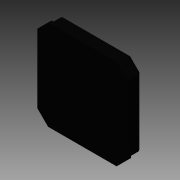
# Autodesk Inventor part: ADAU1761
Saved by Autodesk Inventor 2013 (Build 170138000, 138)
## iProperties
Created: 2015-07-03
Part Number: ADAU1761
Material: Ogólny
Document SubType Name: Modeling
Designer: terg
Density: 1 g/cm^3
Author: terg
Autodesk Inventor part; units mm, degrees
ref_plane "YZ Plane" through (0, 0, 0) normal (1, 0, 0) x (0, 1, 0)
ref_plane "XZ Plane" through (0, 0, 0) normal (0, 1, 0) x (-1, 0, 0)
ref_plane "XY Plane" through (0, 0, 0) normal (0, 0, 1) x (1, 0, 0)
sketch "Szkic1" plane through (0, 0, 0) normal (0, 1, 0) x (-1, 0, 0)
  line L0 (-0.6, 0) -> (-4.4, 0)
  line L1 (-5, -0.6) -> (-5, -4.4)
  line L2 (-4.4, -5) -> (-0.6, -5)
  line L3 (0, -4.4) -> (0, -0.6)
  line L4 (0, -4.4) -> (-0.6, -5)
  line L5 (-4.4, -5) -> (-5, -4.4)
  line L6 (-5, -0.6) -> (-4.4, 0)
  line L7 (-0.6, 0) -> (0, -0.6)
  point P0 (0, 0)
  point P1 (-5, -5)
  point P2 (-5, 0)
  point P3 (0, -5)
  dimension "d0" = 5
  dimension "d1" = 5
  dimension "d2" = 0.6
  dimension "d3" = 0.6
  dimension "d4" = 0.6
  dimension "d5" = 0.6
  dimension "d6" = 0.6
  dimension "d7" = 0.6
  dimension "d8" = 0.6
  dimension "d9" = 0.6
  constraints: 16 end point, 8 point on line, 2 parallel, 1 horizontal, 1 perpendicular
  measures "d0" distance of point (0, -5) point (-5, -5)
  measures "d1" distance of point (-5, -5) point (-5, 0)
  measures "d2" distance of L3.start point (0, -5)
  measures "d3" distance of L2.end point (0, -5)
  measures "d4" distance of L2.start point (-5, -5)
  measures "d5" distance of L1.end point (-5, -5)
  measures "d6" distance of L1.start point (-5, 0)
  measures "d7" distance of L0.end point (-5, 0)
  measures "d8" distance of L0.start point (0, 0)
  measures "d9" distance of L3.end point (0, 0)
extrude "Wyciągnięcie proste1" add sketch "Szkic1" along normal blind 0.2
sketch "Szkic2" plane through (0, 0.2, 0) normal (0, 1, 0) x (1, 0, 0)
  line L0 (0.6, 5) -> (0, 4.4) projected
  line L1 (0, 4.4) -> (0, 0.6) projected
  line L2 (0, 0.6) -> (0.6, 0) projected
  line L3 (0.6, 0) -> (4.4, 0) projected
  line L4 (4.4, 0) -> (5, 0.6) projected
  line L5 (5, 0.6) -> (5, 4.4) projected
  line L6 (5, 4.4) -> (4.4, 5) projected
  line L7 (4.4, 5) -> (0.6, 5) projected
  line L8 (0.6311, 4.925) -> (0.075, 4.3689)
  line L9 (0.075, 4.3689) -> (0.075, 0.6311)
  line L10 (0.075, 0.6311) -> (0.6311, 0.075)
  line L11 (0.6311, 0.075) -> (4.3689, 0.075)
  line L12 (4.3689, 0.075) -> (4.925, 0.6311)
  line L13 (4.925, 0.6311) -> (4.925, 4.3689)
  line L14 (4.925, 4.3689) -> (4.3689, 4.925)
  line L15 (4.3689, 4.925) -> (0.6311, 4.925)
  point P0 (0, 0)
  dimension "d12" = 0.075
  constraints: 16 end point, 7 other
  measures "d12" distance between parallel lines of L7 L15
extrude "Wyciągnięcie proste2" add sketch "Szkic2" along normal blind 0.65 contours L15 L14 L13 L12 L11 L10 L9 L8
fillet "Zaokrąglenie1" radius 0.2 8 edges at (0.075, 0.85, -2.5) (0.353, 0.85, -4.647) (2.5, 0.85, -4.925) (4.647, 0.85, -4.647) (4.925, 0.85, -2.5) (4.647, 0.85, -0.353) (2.5, 0.85, -0.075) (0.353, 0.85, -0.353)
sketch "Szkic3" plane through (0, 0.85, 0) normal (0, 1, 0) x (1, 0, 0)
  line L0 (0.7139, 4.725) -> (4.2861, 4.725) projected
  line L1 (0.275, 0.7139) -> (0.275, 4.2861) projected
  point P0 (0, 0)
  point P1 (0.875, 4.125)
  dimension "d16" = 0.6
  dimension "d17" = 0.6
  measures "d16" distance from line of L0 point (0.875, 4.125)
  measures "d17" distance from line of L1 point (0.875, 4.125)
hole "Otwór1" at (0.875, 0.85, -4.125) direction (0, -1, 0) diameter 0.5 depth 0.1
equation "\"d3\" = d2"
equation "\"d4\" = d2"
equation "\"d5\" = d4"
equation "\"d6\" = d2"
equation "\"d7\" = d6"
equation "\"d8\" = d2"
equation "\"d9\" = d8"
